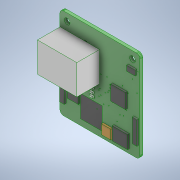
# Autodesk Inventor part: ethernet_poe.brd
Saved by Autodesk Inventor 2020 (Build 240168000, 168)
## iProperties
Created: 2019-12-01
Part Number: ethernet_poe.brd
Material: Generic
Document SubType Name: Modeling
Designer: kylew
Density: 1 g/cm^3
Appearance: Board Outline
Author: kylew
Autodesk Inventor part; units mm, degrees
ref_plane "YZ Plane" through (0, 0, 0) normal (1, 0, 0) x (0, 1, 0)
ref_plane "XZ Plane" through (0, 0, 0) normal (0, 1, 0) x (-1, 0, 0)
ref_plane "XY Plane" through (0, 0, 0) normal (0, 0, 1) x (1, 0, 0)
sketch "Sketch1" plane through (0, 0, 0) normal (0, 0, 1) x (1, 0, 0)
  line L0 (2, 0) -> (42, 0)
  line L1 (42, 0) -> (42.5176, 0.0681)
  line L2 (42.5176, 0.0681) -> (43, 0.2679)
  line L3 (43, 0.2679) -> (43.4142, 0.5858)
  line L4 (43.4142, 0.5858) -> (43.7321, 1)
  line L5 (43.7321, 1) -> (43.9319, 1.4824)
  line L6 (43.9319, 1.4824) -> (44, 2)
  line L7 (44, 2) -> (44, 48)
  line L8 (44, 48) -> (43.9319, 48.5176)
  line L9 (43.9319, 48.5176) -> (43.7321, 49)
  line L10 (43.7321, 49) -> (43.4142, 49.4142)
  line L11 (43.4142, 49.4142) -> (43, 49.7321)
  line L12 (43, 49.7321) -> (42.5176, 49.9319)
  line L13 (42.5176, 49.9319) -> (42, 50)
  line L14 (42, 50) -> (2, 50)
  line L15 (2, 50) -> (1.4824, 49.9319)
  line L16 (1.4824, 49.9319) -> (1, 49.7321)
  line L17 (1, 49.7321) -> (0.5858, 49.4142)
  line L18 (0.5858, 49.4142) -> (0.2679, 49)
  line L19 (0.2679, 49) -> (0.0681, 48.5176)
  line L20 (0.0681, 48.5176) -> (0, 48)
  line L21 (0, 48) -> (0, 2)
  line L22 (0, 2) -> (0.0681, 1.4824)
  line L23 (0.0681, 1.4824) -> (0.2679, 1)
  line L24 (0.2679, 1) -> (0.5858, 0.5858)
  line L25 (0.5858, 0.5858) -> (1, 0.2679)
  line L26 (1, 0.2679) -> (1.4824, 0.0681)
  line L27 (1.4824, 0.0681) -> (2, 0)
  circle A0 centre (26.5, 3.98) radius 0.405
  circle A1 centre (26.5, 6.02) radius 0.405
  circle A2 centre (20, 39) radius 0.45
  circle A3 centre (17.46, 37.73) radius 0.45
  circle A4 centre (20, 36.46) radius 0.45
  circle A5 centre (17.46, 35.19) radius 0.45
  circle A6 centre (20, 33.92) radius 0.45
  circle A7 centre (17.46, 32.65) radius 0.45
  circle A8 centre (20, 28.84) radius 0.45
  circle A9 centre (17.46, 27.57) radius 0.45
  circle A10 centre (6.21, 39.61) radius 0.45
  circle A11 centre (7.73, 37.07) radius 0.45
  circle A12 centre (6.21, 29.5) radius 0.45
  circle A13 centre (7.73, 26.96) radius 0.5
  circle A14 centre (14.16, 41.04) radius 0.85
  circle A15 centre (14.16, 25.54) radius 0.85
  circle A16 centre (2, 18) radius 0.51
  circle A17 centre (2, 15.46) radius 0.51
  circle A18 centre (2, 12.92) radius 0.51
  circle A19 centre (2, 10.38) radius 0.51
  circle A20 centre (2, 7.84) radius 0.51
  circle A21 centre (42, 18) radius 0.51
  circle A22 centre (42, 15.46) radius 0.51
  circle A23 centre (42, 12.92) radius 0.51
  circle A24 centre (42, 10.38) radius 0.51
  circle A25 centre (42, 7.84) radius 0.51
  circle A26 centre (40, 46) radius 1.575
  circle A27 centre (4, 46) radius 1.575
  circle A28 centre (11.11, 27.57) radius 1.6
  circle A29 centre (11.11, 39) radius 1.6
  circle A30 centre (36.5, 20) radius 0.2032
  circle A31 centre (33.5, 22.5) radius 0.2032
  circle A32 centre (6.5, 18.5) radius 0.2032
  circle A33 centre (22.5, 20) radius 0.2032
  circle A34 centre (4.5, 16.5) radius 0.2032
  circle A35 centre (33.5, 28) radius 0.2032
  circle A36 centre (32.5, 28) radius 0.2032
  circle A37 centre (32.5, 27) radius 0.2032
  circle A38 centre (26.5, 23.5) radius 0.2032
  circle A39 centre (36, 25.5) radius 0.2032
  circle A40 centre (24.1, 16.5) radius 0.2032
  circle A41 centre (3.5, 21.5) radius 0.2032
  circle A42 centre (3.5, 14.5) radius 0.2032
  circle A43 centre (10.5, 10.5) radius 0.2032
  circle A44 centre (10.5, 9.5) radius 0.2032
  circle A45 centre (20.5, 12.5) radius 0.2032
  circle A46 centre (21.5, 19) radius 0.2032
  circle A47 centre (19, 17) radius 0.2032
  circle A48 centre (8.5, 22.5) radius 0.2032
  circle A49 centre (21.5, 22) radius 0.2032
  circle A50 centre (29, 20) radius 0.2032
  circle A51 centre (27.5, 26) radius 0.2032
  circle A52 centre (37.5, 28.5) radius 0.2032
  circle A53 centre (34.5, 30.5) radius 0.2032
  circle A54 centre (32.5, 22) radius 0.2032
  circle A55 centre (31.4, 27.3) radius 0.2032
  circle A56 centre (5.2, 19) radius 0.2032
  circle A57 centre (31, 7) radius 0.2032
  circle A58 centre (5.1, 9.5) radius 0.2032
  circle A59 centre (42.5, 31) radius 0.2032
  circle A60 centre (43, 41.5) radius 0.2032
  circle A61 centre (14, 22) radius 0.2032
  circle A62 centre (14, 19.5) radius 0.2032
  circle A63 centre (16, 23) radius 0.2032
  circle A64 centre (33, 16) radius 0.2032
  circle A65 centre (35, 16.5) radius 0.2032
  circle A66 centre (40, 36.5) radius 0.2032
  circle A67 centre (31.5, 12) radius 0.2032
  circle A68 centre (22.5, 30) radius 0.2032
  circle A69 centre (26, 30.5) radius 0.2032
  circle A70 centre (27.5, 27.5) radius 0.2032
  circle A71 centre (26.9, 17.3) radius 0.2032
  circle A72 centre (15, 32.5) radius 0.2032
  circle A73 centre (22, 23) radius 0.2032
  circle A74 centre (25, 22.5) radius 0.2032
  circle A75 centre (30, 22.5) radius 0.2032
  circle A76 centre (30.5, 23.5) radius 0.2032
  circle A77 centre (27, 24.5) radius 0.2032
  circle A78 centre (30.6, 27.7) radius 0.2032
  circle A79 centre (21.5, 38.5) radius 0.2032
  constraints: 80 centre point, 56 end point
extrude "ethernet_poe.brd_Outline" add sketch "Sketch1" along normal blind 1.6
sketch "E2-5, E2-5_1" plane through (0, 0, 1.6) normal (0, 0, 1) x (1, 0, 0)
  line L0 (23.8838, 2.3838) -> (23.8838, 7.6162)
  line L1 (23.8838, 7.6162) -> (29.1162, 7.6162)
  line L2 (29.1162, 7.6162) -> (29.1162, 2.3838)
  line L3 (29.1162, 2.3838) -> (23.8838, 2.3838)
  constraints: 8 end point
extrude "C20_2" add sketch "E2-5, E2-5_1" along normal blind 1
sketch "CHIP-LED0603, CHIP-LED0603_3" plane through (0, 0, 1.6) normal (0, 0, 1) x (1, 0, 0)
  line L0 (17.15, 21.0492) -> (17.15, 21.95)
  line L1 (17.15, 21.95) -> (18.85, 21.95)
  line L2 (18.85, 21.95) -> (18.85, 21.0492)
  line L3 (18.85, 21.0492) -> (17.15, 21.0492)
  constraints: 8 end point
extrude "D2_4" add sketch "CHIP-LED0603, CHIP-LED0603_3" along normal blind 1
sketch "CHIP-LED0603, CHIP-LED0603_5" plane through (0, 0, 1.6) normal (0, 0, 1) x (1, 0, 0)
  line L0 (17.15, 17.1492) -> (17.15, 18.05)
  line L1 (17.15, 18.05) -> (18.85, 18.05)
  line L2 (18.85, 18.05) -> (18.85, 17.1492)
  line L3 (18.85, 17.1492) -> (17.15, 17.1492)
  constraints: 8 end point
extrude "D3_6" add sketch "CHIP-LED0603, CHIP-LED0603_5" along normal blind 1
sketch "CHIP-LED0603, CHIP-LED0603_7" plane through (0, 0, 1.6) normal (0, 0, 1) x (1, 0, 0)
  line L0 (17.15, 19.0492) -> (17.15, 19.95)
  line L1 (17.15, 19.95) -> (18.85, 19.95)
  line L2 (18.85, 19.95) -> (18.85, 19.0492)
  line L3 (18.85, 19.0492) -> (17.15, 19.0492)
  constraints: 8 end point
extrude "D4_8" add sketch "CHIP-LED0603, CHIP-LED0603_7" along normal blind 1
sketch "ARJP11A-MBSB-A-B-EMU2, ARJP11A_9" plane through (0, 0, 1.6) normal (0, 0, 1) x (1, 0, 0)
  line L0 (21.8, 41.4785) -> (21.8, 25.0915)
  line L1 (21.8, 25.0915) -> (0.1465, 25.0915)
  line L2 (0.1465, 25.0915) -> (0.1465, 41.4785)
  line L3 (0.1465, 41.4785) -> (21.8, 41.4785)
  constraints: 8 end point
extrude "J1_10" add sketch "ARJP11A-MBSB-A-B-EMU2, ARJP11A_9" along normal blind 12.5
sketch "1X05, J2_1X05_11" plane through (0, 0, 1.6) normal (0, 0, 1) x (1, 0, 0)
  line L0 (3.3716, 19.27) -> (3.3716, 6.57)
  line L1 (3.3716, 6.57) -> (0.73, 6.57)
  line L2 (0.73, 6.57) -> (0.73, 19.27)
  line L3 (0.73, 19.27) -> (3.3716, 19.27)
  constraints: 8 end point
extrude "J2_12" add sketch "1X05, J2_1X05_11" along normal blind 1
sketch "1X05, J3_1X05_13" plane through (0, 0, 1.6) normal (0, 0, 1) x (1, 0, 0)
  line L0 (43.3716, 19.27) -> (43.3716, 6.57)
  line L1 (43.3716, 6.57) -> (40.73, 6.57)
  line L2 (40.73, 6.57) -> (40.73, 19.27)
  line L3 (40.73, 19.27) -> (43.3716, 19.27)
  constraints: 8 end point
extrude "J3_14" add sketch "1X05, J3_1X05_13" along normal blind 1
sketch "744771147, 47_15" plane through (0, 0, 1.6) normal (0, 0, 1) x (1, 0, 0)
  line L0 (23.3, 3.2365) -> (11.2365, 3.2365)
  line L1 (11.2365, 3.2365) -> (11.2365, 15.3635)
  line L2 (11.2365, 15.3635) -> (23.3, 15.3635)
  line L3 (23.3, 15.3635) -> (23.3, 3.2365)
  constraints: 8 end point
extrude "UH_16" add sketch "744771147, 47_15" along normal blind 0.01
sketch "KMR2, KMR2_17" plane through (0, 0, 1.6) normal (0, 0, 1) x (1, 0, 0)
  line L0 (37.6365, 42.4635) -> (42.3635, 42.4635)
  line L1 (42.3635, 42.4635) -> (42.3635, 39.6)
  line L2 (42.3635, 39.6) -> (37.6365, 39.6)
  line L3 (37.6365, 39.6) -> (37.6365, 42.4635)
  constraints: 8 end point
extrude "S1_18" add sketch "KMR2, KMR2_17" along normal blind 1
sketch "48-LQFP, W5500_21" plane through (0, 0, 1.6) normal (0, 0, 1) x (1, 0, 0)
  line L0 (37.1275, 29.1275) -> (37.1275, 20.925)
  line L1 (37.1275, 20.925) -> (28.925, 20.925)
  line L2 (28.925, 20.925) -> (28.925, 29.1275)
  line L3 (28.925, 29.1275) -> (37.1275, 29.1275)
  constraints: 8 end point
extrude "U1_22" add sketch "48-LQFP, W5500_21" along normal blind 1
sketch "SOIC-8-EXPOSED_PAD, IFX91041_23" plane through (0, 0, 1.6) normal (0, 0, 1) x (1, 0, 0)
  line L0 (5, 10.4) -> (5, 17.6)
  line L1 (5, 17.6) -> (11, 17.6)
  line L2 (11, 17.6) -> (11, 10.4)
  line L3 (11, 10.4) -> (5, 10.4)
  constraints: 8 end point
extrude "U2_24" add sketch "SOIC-8-EXPOSED_PAD, IFX91041_23" along normal blind 1
sketch "SOT230P700X180-4N, AZ1117EH-3_3TRG1_25" plane through (0, 0, 1.6) normal (0, 0, 1) x (1, 0, 0)
  line L0 (29.74, 9.625) -> (38.26, 9.625)
  line L1 (38.26, 9.625) -> (38.26, 2.4)
  line L2 (38.26, 2.4) -> (29.74, 2.4)
  line L3 (29.74, 2.4) -> (29.74, 9.625)
  constraints: 8 end point
extrude "U3_26" add sketch "SOT230P700X180-4N, AZ1117EH-3_3TRG1_25" along normal blind 1
body "Solid1"
